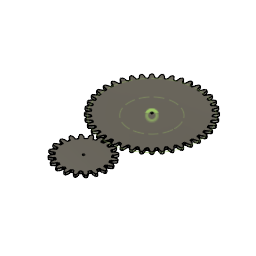
first gears (Autodesk Fusion 360 design; units mm, degrees)
part number: 2026-04-20-18-38-35-079
Autodesk Fusion 360 part; units mm, degrees
sketch "Base Circle" plane through (0, 0, 0) normal (0, 0, 1) x (1, 0, 0)
  circle A0 centre (0, 0) radius 88.43
  circle A1 centre (0, 0) radius 4
extrude "Extrude1" add sketch "Base Circle" along normal blind 10 makes body 1
sketch "Gear Tooth" plane through (0, 0, 0) normal (0, 0, 1) x (1, 0, 0)
  spline S0 degree 5 poles (93.5593, -8.7681) (93.6068, -8.7726) (93.7017, -8.7802) (93.8443, -8.7878) (94.0346, -8.7906) (94.2728, -8.7843) (94.5112, -8.7708) (94.7498, -8.753) (94.9884, -8.7329) (95.2271, -8.7112) (95.4658, -8.6878) (95.7044, -8.6621) (95.943, -8.6335) (96.1816, -8.6013) (96.4202, -8.5657) (96.6587, -8.527) (96.8971, -8.4855) (97.1354, -8.4417) (97.3737, -8.396) (97.6118, -8.3485) (97.8498, -8.299) (98.0877, -8.2476) (98.3255, -8.1941) (98.5631, -8.1384) (98.8007, -8.0806) (99.038, -8.0208) (99.2752, -7.9591) (99.5123, -7.8955) (99.7492, -7.8302) (99.9859, -7.7632) (100.2225, -7.6945) (100.4588, -7.6241) (100.695, -7.552) (100.931, -7.4782) (101.1668, -7.4027) (101.4024, -7.3255) (101.6378, -7.2468) (101.873, -7.1665) (102.108, -7.0846) (102.3428, -7.0012) (102.5773, -6.9163) (102.8116, -6.8298) (103.0457, -6.7419) (103.2796, -6.6525) (103.5132, -6.5616) (103.7466, -6.4693) (103.9797, -6.3756) (104.2126, -6.2804) (104.4453, -6.1838) (104.6777, -6.0859) (104.9098, -5.9865) (105.1417, -5.8858) (105.3733, -5.7838) (105.6047, -5.6804) (105.8357, -5.5757) (106.0665, -5.4696) (106.2971, -5.3622) (106.5273, -5.2536) (106.7573, -5.1436) (106.9869, -5.0324) (107.2163, -4.9199) (107.4454, -4.8062) (107.6742, -4.6912) (107.9027, -4.5749) (108.1309, -4.4574) (108.3588, -4.3387) (108.5864, -4.2188) (108.8136, -4.0977) (109.0406, -3.9753) (109.2672, -3.8518) (109.4935, -3.7271) (109.6743, -3.6264) (109.8098, -3.5503) (109.9, -3.4994) (109.9451, -3.4738) knots 0 0 0 0 0 0 0.01428571 0.02857143 0.04285714 0.05714286 0.07142857 0.08571429 0.1 0.11428571 0.12857143 0.14285714 0.15714286 0.17142857 0.18571429 0.2 0.21428571 0.22857143 0.24285714 0.25714286 0.27142857 0.28571429 0.3 0.31428571 0.32857143 0.34285714 0.35714286 0.37142857 0.38571429 0.4 0.41428571 0.42857143 0.44285714 0.45714286 0.47142857 0.48571429 0.5 0.51428571 0.52857143 0.54285714 0.55714286 0.57142857 0.58571429 0.6 0.61428571 0.62857143 0.64285714 0.65714286 0.67142857 0.68571429 0.7 0.71428571 0.72857143 0.74285714 0.75714286 0.77142857 0.78571429 0.8 0.81428571 0.82857143 0.84285714 0.85714286 0.87142857 0.88571429 0.9 0.91428571 0.92857143 0.94285714 0.95714286 0.97142857 0.98571429 1 1 1 1 1 1
  spline S1 degree 5 poles (93.5593, 8.7681) (93.6068, 8.7726) (93.7017, 8.7802) (93.8443, 8.7878) (94.0346, 8.7906) (94.2728, 8.7843) (94.5112, 8.7708) (94.7498, 8.753) (94.9884, 8.7329) (95.2271, 8.7112) (95.4658, 8.6878) (95.7044, 8.6621) (95.943, 8.6335) (96.1816, 8.6013) (96.4202, 8.5657) (96.6587, 8.527) (96.8971, 8.4855) (97.1354, 8.4417) (97.3737, 8.396) (97.6118, 8.3485) (97.8498, 8.299) (98.0877, 8.2476) (98.3255, 8.1941) (98.5631, 8.1384) (98.8007, 8.0806) (99.038, 8.0208) (99.2752, 7.9591) (99.5123, 7.8955) (99.7492, 7.8302) (99.9859, 7.7632) (100.2225, 7.6945) (100.4588, 7.6241) (100.695, 7.552) (100.931, 7.4782) (101.1668, 7.4027) (101.4024, 7.3255) (101.6378, 7.2468) (101.873, 7.1665) (102.108, 7.0846) (102.3428, 7.0012) (102.5773, 6.9163) (102.8116, 6.8298) (103.0457, 6.7419) (103.2796, 6.6525) (103.5132, 6.5616) (103.7466, 6.4693) (103.9797, 6.3756) (104.2126, 6.2804) (104.4453, 6.1838) (104.6777, 6.0859) (104.9098, 5.9865) (105.1417, 5.8858) (105.3733, 5.7838) (105.6047, 5.6804) (105.8357, 5.5757) (106.0665, 5.4696) (106.2971, 5.3622) (106.5273, 5.2536) (106.7573, 5.1436) (106.9869, 5.0324) (107.2163, 4.9199) (107.4454, 4.8062) (107.6742, 4.6912) (107.9027, 4.5749) (108.1309, 4.4574) (108.3588, 4.3387) (108.5864, 4.2188) (108.8136, 4.0977) (109.0406, 3.9753) (109.2672, 3.8518) (109.4935, 3.7271) (109.6743, 3.6264) (109.8098, 3.5503) (109.9, 3.4994) (109.9451, 3.4738) knots 0 0 0 0 0 0 0.01428571 0.02857143 0.04285714 0.05714286 0.07142857 0.08571429 0.1 0.11428571 0.12857143 0.14285714 0.15714286 0.17142857 0.18571429 0.2 0.21428571 0.22857143 0.24285714 0.25714286 0.27142857 0.28571429 0.3 0.31428571 0.32857143 0.34285714 0.35714286 0.37142857 0.38571429 0.4 0.41428571 0.42857143 0.44285714 0.45714286 0.47142857 0.48571429 0.5 0.51428571 0.52857143 0.54285714 0.55714286 0.57142857 0.58571429 0.6 0.61428571 0.62857143 0.64285714 0.65714286 0.67142857 0.68571429 0.7 0.71428571 0.72857143 0.74285714 0.75714286 0.77142857 0.78571429 0.8 0.81428571 0.82857143 0.84285714 0.85714286 0.87142857 0.88571429 0.9 0.91428571 0.92857143 0.94285714 0.95714286 0.97142857 0.98571429 1 1 1 1 1 1
  arc A0 (109.9451, -3.4738) -> (109.9451, 3.4738) centre (0, 0) ccw
  line L0 (88.0342, -8.2503) -> (93.5593, -8.7681)
  line L1 (88.0342, 8.2503) -> (93.5593, 8.7681)
  line L2 (88.0342, -8.2503) -> (88.0342, 8.2503)
  point P0 (94.7105, -8.7555)
  point P1 (95.8707, -8.6417)
  point P2 (97.0364, -8.4596)
  point P3 (98.206, -8.2207)
  point P4 (99.3785, -7.9312)
  point P5 (100.5531, -7.5951)
  point P6 (101.7291, -7.2154)
  point P7 (102.9056, -6.7943)
  point P8 (104.0822, -6.3335)
  point P9 (105.2582, -5.8343)
  point P10 (106.4331, -5.2979)
  point P11 (107.6062, -4.7251)
  point P12 (108.7771, -4.1169)
  point P13 (94.7105, 8.7555)
  point P14 (95.8707, 8.6417)
  point P15 (97.0364, 8.4596)
  point P16 (98.206, 8.2207)
  point P17 (99.3785, 7.9312)
  point P18 (100.5531, 7.5951)
  point P19 (101.7291, 7.2154)
  point P20 (102.9056, 6.7943)
  point P21 (104.0822, 6.3335)
  point P22 (105.2582, 5.8343)
  point P23 (106.4331, 5.2979)
  point P24 (107.6062, 4.7251)
  point P25 (108.7771, 4.1169)
extrude "Extrude2" add sketch "Gear Tooth" along normal blind 10 bodies 1
fillet "Fillet1" radius 2 2 edges at (88.0442, -8.2513, 5) (88.0442, 8.2513, 5) on bodies 1
pattern_circular "C-Pattern1" count 20 over 360 about axis through (0, 0, 0) along (0, 0, 1) of "Extrude2", "Fillet1"
sketch "Diametrial Pitch Circle" plane through (0, 0, 0) normal (0, 0, 1) x (1, 0, 0)
  circle A0 centre (0, 0) radius 100 construction
sketch "Base Circle (1)" plane through (0, 0, 0) normal (0, 0, 1) x (1, 0, 0)
  circle A0 centre (0, 0) radius 188.43
  circle A1 centre (0, 0) radius 4
extrude "Extrude3" add sketch "Base Circle (1)" along normal blind 10 separate body makes body 2
sketch "Gear Tooth (1)" plane through (0, 0, 0) normal (0, 0, 1) x (1, 0, 0)
  spline S0 degree 5 poles (187.6628, -10.1765) (187.7276, -10.177) (187.8571, -10.1776) (188.0514, -10.1767) (188.3106, -10.1724) (188.6345, -10.1615) (188.9584, -10.1452) (189.2823, -10.1237) (189.6063, -10.0973) (189.9302, -10.0663) (190.2541, -10.0312) (190.5778, -9.9925) (190.9015, -9.9506) (191.2251, -9.9059) (191.5486, -9.8585) (191.8719, -9.8084) (192.1951, -9.7558) (192.5181, -9.7005) (192.841, -9.6427) (193.1638, -9.5823) (193.4864, -9.5194) (193.8088, -9.4542) (194.1311, -9.3867) (194.4532, -9.3171) (194.7752, -9.2453) (195.097, -9.1715) (195.4185, -9.0956) (195.7399, -9.0177) (196.0612, -8.9378) (196.3822, -8.856) (196.703, -8.7722) (197.0236, -8.6865) (197.3441, -8.5989) (197.6643, -8.5096) (197.9843, -8.4184) (198.3041, -8.3255) (198.6237, -8.2308) (198.9431, -8.1344) (199.2622, -8.0363) (199.5811, -7.9365) (199.8999, -7.8351) (200.2183, -7.732) (200.5366, -7.6273) (200.8546, -7.5209) (201.1724, -7.413) (201.4899, -7.3035) (201.8072, -7.1925) (202.1243, -7.0799) (202.4411, -6.9658) (202.7577, -6.8502) (203.074, -6.7331) (203.3901, -6.6146) (203.7059, -6.4945) (204.0214, -6.373) (204.3367, -6.2501) (204.6518, -6.1257) (204.9666, -5.9999) (205.2811, -5.8728) (205.5953, -5.7442) (205.9093, -5.6142) (206.223, -5.4829) (206.5364, -5.3502) (206.8496, -5.2161) (207.1625, -5.0808) (207.4751, -4.944) (207.7874, -4.806) (208.0994, -4.6666) (208.4112, -4.526) (208.7227, -4.384) (209.0338, -4.2408) (209.3447, -4.0963) (209.5932, -3.9797) (209.7794, -3.8916) (209.9035, -3.8327) (209.9656, -3.8031) knots 0 0 0 0 0 0 0.01428571 0.02857143 0.04285714 0.05714286 0.07142857 0.08571429 0.1 0.11428571 0.12857143 0.14285714 0.15714286 0.17142857 0.18571429 0.2 0.21428571 0.22857143 0.24285714 0.25714286 0.27142857 0.28571429 0.3 0.31428571 0.32857143 0.34285714 0.35714286 0.37142857 0.38571429 0.4 0.41428571 0.42857143 0.44285714 0.45714286 0.47142857 0.48571429 0.5 0.51428571 0.52857143 0.54285714 0.55714286 0.57142857 0.58571429 0.6 0.61428571 0.62857143 0.64285714 0.65714286 0.67142857 0.68571429 0.7 0.71428571 0.72857143 0.74285714 0.75714286 0.77142857 0.78571429 0.8 0.81428571 0.82857143 0.84285714 0.85714286 0.87142857 0.88571429 0.9 0.91428571 0.92857143 0.94285714 0.95714286 0.97142857 0.98571429 1 1 1 1 1 1
  spline S1 degree 5 poles (187.6628, 10.1765) (187.7276, 10.177) (187.8571, 10.1776) (188.0514, 10.1767) (188.3106, 10.1724) (188.6345, 10.1615) (188.9584, 10.1452) (189.2823, 10.1237) (189.6063, 10.0973) (189.9302, 10.0663) (190.2541, 10.0312) (190.5778, 9.9925) (190.9015, 9.9506) (191.2251, 9.9059) (191.5486, 9.8585) (191.8719, 9.8084) (192.1951, 9.7558) (192.5181, 9.7005) (192.841, 9.6427) (193.1638, 9.5823) (193.4864, 9.5194) (193.8088, 9.4542) (194.1311, 9.3867) (194.4532, 9.3171) (194.7752, 9.2453) (195.097, 9.1715) (195.4185, 9.0956) (195.7399, 9.0177) (196.0612, 8.9378) (196.3822, 8.856) (196.703, 8.7722) (197.0236, 8.6865) (197.3441, 8.5989) (197.6643, 8.5096) (197.9843, 8.4184) (198.3041, 8.3255) (198.6237, 8.2308) (198.9431, 8.1344) (199.2622, 8.0363) (199.5811, 7.9365) (199.8999, 7.8351) (200.2183, 7.732) (200.5366, 7.6273) (200.8546, 7.5209) (201.1724, 7.413) (201.4899, 7.3035) (201.8072, 7.1925) (202.1243, 7.0799) (202.4411, 6.9658) (202.7577, 6.8502) (203.074, 6.7331) (203.3901, 6.6146) (203.7059, 6.4945) (204.0214, 6.373) (204.3367, 6.2501) (204.6518, 6.1257) (204.9666, 5.9999) (205.2811, 5.8728) (205.5953, 5.7442) (205.9093, 5.6142) (206.223, 5.4829) (206.5364, 5.3502) (206.8496, 5.2161) (207.1625, 5.0808) (207.4751, 4.944) (207.7874, 4.806) (208.0994, 4.6666) (208.4112, 4.526) (208.7227, 4.384) (209.0338, 4.2408) (209.3447, 4.0963) (209.5932, 3.9797) (209.7794, 3.8916) (209.9035, 3.8327) (209.9656, 3.8031) knots 0 0 0 0 0 0 0.01428571 0.02857143 0.04285714 0.05714286 0.07142857 0.08571429 0.1 0.11428571 0.12857143 0.14285714 0.15714286 0.17142857 0.18571429 0.2 0.21428571 0.22857143 0.24285714 0.25714286 0.27142857 0.28571429 0.3 0.31428571 0.32857143 0.34285714 0.35714286 0.37142857 0.38571429 0.4 0.41428571 0.42857143 0.44285714 0.45714286 0.47142857 0.48571429 0.5 0.51428571 0.52857143 0.54285714 0.55714286 0.57142857 0.58571429 0.6 0.61428571 0.62857143 0.64285714 0.65714286 0.67142857 0.68571429 0.7 0.71428571 0.72857143 0.74285714 0.75714286 0.77142857 0.78571429 0.8 0.81428571 0.82857143 0.84285714 0.85714286 0.87142857 0.88571429 0.9 0.91428571 0.92857143 0.94285714 0.95714286 0.97142857 0.98571429 1 1 1 1 1 1
  arc A0 (209.9656, -3.8031) -> (209.9656, 3.8031) centre (0, 0) ccw
  line L0 (187.6628, 10.1765) -> (187.6628, -10.1765)
  point P0 (189.2437, -10.1253)
  point P1 (190.8305, -9.9593)
  point P2 (192.4208, -9.7168)
  point P3 (194.0137, -9.411)
  point P4 (195.6084, -9.0494)
  point P5 (197.2044, -8.6369)
  point P6 (198.8012, -8.177)
  point P7 (200.3983, -7.6726)
  point P8 (201.9953, -7.1255)
  point P9 (203.5918, -6.5377)
  point P10 (205.1874, -5.9104)
  point P11 (206.7819, -5.2449)
  point P12 (208.3747, -4.5422)
  point P13 (189.2437, 10.1253)
  point P14 (190.8305, 9.9593)
  point P15 (192.4208, 9.7168)
  point P16 (194.0137, 9.411)
  point P17 (195.6084, 9.0494)
  point P18 (197.2044, 8.6369)
  point P19 (198.8012, 8.177)
  point P20 (200.3983, 7.6726)
  point P21 (201.9953, 7.1255)
  point P22 (203.5918, 6.5377)
  point P23 (205.1874, 5.9104)
  point P24 (206.7819, 5.2449)
  point P25 (208.3747, 4.5422)
extrude "Extrude4" add sketch "Gear Tooth (1)" along normal blind 10 bodies 2
fillet "Fillet2" radius 2 2 edges at (188.1551, 10.1743, 5) (188.1551, -10.1743, 5) on bodies 2
pattern_circular "C-Pattern2" count 40 over 360 about axis through (0, 0, 0) along (0, 0, 1) of "Extrude4", "Fillet2"
sketch "Diametrial Pitch Circle (1)" plane through (0, 0, 0) normal (0, 0, 1) x (1, 0, 0)
  circle A0 centre (0, 0) radius 200 construction
move_body "Move1" bodies 1 to x (1, 0, 0) y (0, 1, 0) z (0, 0, 1) at (0, -300, 0)
move_body "Move2" bodies 1 to x (0.996195, -0.087156, 0) y (0.087156, 0.996195, 0) z (0, 0, 1) at (35.3153, -11.1473, 0)
named bodies: "Spur Gear (20 teeth)", "Spur Gear (40 teeth)"
